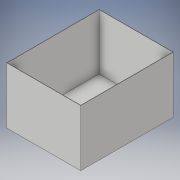
# Autodesk Inventor part: 563-AU1028MG-PE4312
Saved by Autodesk Inventor 2018 (Build 220112000, 112)
## iProperties
Created: 2018-04-30
Part Number: 563-AU1028MG-PE4312
Material: Generic
Document SubType Name: Modeling
Designer: bbramman
Density: 1 g/cm^3
Appearance: Default
Author: bbramman
Autodesk Inventor part; units mm, degrees
ref_plane "YZ Plane" through (0, 0, 0) normal (1, 0, 0) x (0, 1, 0)
ref_plane "XZ Plane" through (0, 0, 0) normal (0, 1, 0) x (-1, 0, 0)
ref_plane "XY Plane" through (0, 0, 0) normal (0, 0, 1) x (1, 0, 0)
sketch "Sketch1" plane through (0, 0, 0) normal (0, 1, 0) x (-1, 0, 0)
  line L0 (-50.8, 63.5) -> (50.8, 63.5)
  line L1 (50.8, 63.5) -> (50.8, -63.5)
  line L2 (50.8, -63.5) -> (-50.8, -63.5)
  line L3 (-50.8, -63.5) -> (-50.8, 63.5)
  line L4 (-50.8, 63.5) -> (50.8, -63.5) construction
  line L5 (50.8, 63.5) -> (-50.8, -63.5) construction
  point P0 (0, 0)
  dimension "d0" = 101.6
  dimension "d1" = 127
  constraints: 12 end point, 2 midpoint, 2 parallel, 1 horizontal, 1 perpendicular
  measures "d0" distance of L1.end L2.end
  measures "d1" distance of L0.end L1.end
extrude "Extrusion1" add sketch "Sketch1" along normal blind 1.016
sketch "Sketch2" plane through (0, 1.016, 0) normal (0, 1, 0) x (1, 0, 0)
  line L0 (50.8, 63.5) -> (-50.8, 63.5) projected
  line L1 (50.8, -63.5) -> (-50.8, -63.5)
  line L2 (-50.8, -63.5) -> (-50.8, 63.5)
  line L3 (-50.8, 63.5) -> (50.8, 63.5)
  line L4 (50.8, 63.5) -> (50.8, -63.5)
  line L5 (50.8, -63.5) -> (-50.8, 63.5) construction
  line L6 (-50.8, -63.5) -> (50.8, 63.5) construction
  line L7 (50.292, -62.992) -> (-50.292, -62.992)
  line L8 (-50.292, -62.992) -> (-50.292, 62.992)
  line L9 (-50.292, 62.992) -> (50.292, 62.992)
  line L10 (50.292, 62.992) -> (50.292, -62.992)
  line L11 (50.292, -62.992) -> (-50.292, 62.992) construction
  line L12 (-50.292, -62.992) -> (50.292, 62.992) construction
  point P0 (0, 0)
  dimension "d4" = 100.584
  dimension "d5" = 125.984
  constraints: 24 end point, 4 midpoint, 4 parallel, 2 horizontal, 2 perpendicular
  measures "d4" distance of L8.end L9.end
  measures "d5" distance of L7.end L8.end
extrude "Extrusion2" add sketch "Sketch2" along normal blind 76.2
sketch "Sketch3" plane through (0, 1.016, 0) normal (0, 1, 0) x (1, 0, 0)
  line L0 (0, 0) -> (0, -25.4)
  line L1 (0, -25.4) -> (0, 25.4)
  circle A0 centre (0, -25.4) radius 2.0828
  circle A1 centre (0, 25.4) radius 2.0828
  dimension "d8" = 25.4
  dimension "d9" = 50.8
  dimension "d10" = 4.1656
  dimension "d11" = 4.1656
  constraints: 4 end point, 2 centre point, 2 coincident, 1 point on line, 1 vertical
  measures "d8" distance of L0.start L0.end
  measures "d9" distance of L0.end L1.end
  measures "d10" diameter of A0
  measures "d11" diameter of A1
extrude "Extrusion3" cut sketch "Sketch3" against normal through all
body "Solid1"
